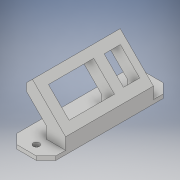
# Autodesk Inventor part: Indicator
Saved by Autodesk Inventor 2019.4 (Build 234330000, 330)
## iProperties
Created: 2020-04-10
Part Number: Indicator
Material: Типовые
Document SubType Name: Modeling
Designer: NoName
Density: 1 g/cm^3
Appearance: По умолчанию
Author: NoName
Autodesk Inventor part; units mm, degrees
ref_plane "YZ Plane" through (0, 0, 0) normal (1, 0, 0) x (0, 1, 0)
ref_plane "XZ Plane" through (0, 0, 0) normal (0, 1, 0) x (-1, 0, 0)
ref_plane "XY Plane" through (0, 0, 0) normal (0, 0, 1) x (1, 0, 0)
sketch "Эскиз1" plane through (0, 0, 0) normal (0, 0, 1) x (1, 0, 0)
  line L0 (-10, 0) -> (10, 0)
  line L1 (-10, 25) -> (-10, 0)
  line L2 (-10, 25) -> (-7, 25)
  line L3 (-7, 25) -> (10, 8)
  line L4 (10, 8) -> (10, 0)
  point P0 (0, 0)
  point P1 (0, 0)
  dimension "d4" = 20
  dimension "d5" = 25
  dimension "d6" = 3
  dimension "d7" = 135
  constraints: 10 end point, 2 horizontal, 1 coincident, 1 midpoint, 1 perpendicular
  measures "d4" distance of L0.start L0.end
  measures "d5" distance of L1.start L0.start
  measures "d6" distance of L1.start L2.end
  measures "d7" angle of L4 L3
extrude "Выдавливание1" add sketch "Эскиз1" along normal mid plane 45
sketch "Эскиз3" plane through (-7, 25, -22.5) normal (0.7071, 0.7071, 0) x (-0.7071, 0.7071, 0)
  line L0 (-4.5208, 40) -> (-19.5208, 40)
  line L1 (-19.5208, 40) -> (-19.5208, 16.8)
  line L2 (-19.5208, 16.8) -> (-4.5208, 16.8)
  line L3 (-4.5208, 16.8) -> (-4.5208, 40)
  line L4 (-24.0416, 45) -> (0, 45) projected
  line L5 (-5.0208, 11.8) -> (-19.0208, 11.8)
  line L6 (-19.0208, 11.8) -> (-19.0208, 3.5)
  line L7 (-19.0208, 3.5) -> (-5.0208, 3.5)
  line L8 (-5.0208, 3.5) -> (-5.0208, 11.8)
  line L9 (0, 0) -> (-24.0416, 0) projected
  point P0 (-22.6274, 22.5)
  point P1 (-12.0208, 11.8)
  point P2 (-12.0208, 16.8)
  point P3 (-12.0208, 3.5)
  point P4 (-12.0208, 0)
  dimension "d8" = 23.2
  dimension "d9" = 15
  dimension "d10" = 5
  dimension "d11" = 14
  dimension "d12" = 8.3
  dimension "d13" = 5
  constraints: 16 end point, 4 midpoint, 4 parallel, 2 horizontal, 2 perpendicular, 2 vertical alignment
  measures "d8" distance between parallel lines of L2 L0
  measures "d9" distance between parallel lines of L1 L3
  measures "d10" distance between parallel lines of L4 L0
  measures "d11" distance of L6.end L7.end
  measures "d12" distance of L7.end L5.start
  measures "d13" distance between parallel lines of L2 L5
extrude "Выдавливание2" cut sketch "Эскиз3" against normal blind 10
sketch "Эскиз7" plane through (0, 0, 22.5) normal (0, 0, 1) x (1, 0, 0)
  line L0 (10, 0) -> (-10, 0) projected
  line L1 (0, 8.1005) -> (-10, 18.1005)
  line L2 (10, 8) -> (-7, 25) projected
  line L3 (6.8033, 11.1967) -> (-3.8033, 21.8033) projected
  line L4 (10, 8) -> (10, 0) projected
  line L5 (-7, 25) -> (10, 8)
  line L6 (-7, 25) -> (10, 8) projected
  line L7 (0, 8.1005) -> (0, 2)
  line L8 (0, 2) -> (-10, 2)
  line L9 (-10, 2) -> (-10, 0)
  line L10 (-10, 0) -> (10, 0)
  line L11 (10, 8) -> (10, 0)
  line L12 (-10, 18.1005) -> (-10, 22)
  line L13 (-10, 22) -> (-7, 25)
  line L14 (-10, 25) -> (-10, 0) projected
  point P0 (0, 0)
  point P1 (1.5, 16.5)
  dimension "d22" = 7
  dimension "d24" = 2
  dimension "d25" = 10
  dimension "d26" = 135
  constraints: 18 end point, 3 vertical, 2 collinear, 1 midpoint, 1 parallel, 1 point on line
  measures "d22" distance between parallel lines of L2 L1
  measures "d24" distance between parallel lines of L0 L8
  measures "d25" distance between parallel lines of L4 L7
  measures "d26" angle of L12 L13
extrude "Выдавливание4" cut sketch "Эскиз7" against normal through all contours L0 L9 L8 L7 L1 L12 L13 L2 L4 keep common part
sketch "Эскиз8" plane through (0, 0, -22.5) normal (0, 0, -1) x (-1, 0, 0)
  line L0 (10, 2) -> (0, 2) projected
  line L1 (-10, 0) -> (10, 0) projected
  line L2 (10, 2) -> (-10, 2)
  line L3 (-10, 2) -> (-10, 0)
  line L4 (-10, 0) -> (10, 0)
  line L5 (10, 0) -> (10, 2)
  point P0 (0, 0)
  constraints: 8 end point, 2 parallel, 1 horizontal, 1 perpendicular
extrude "Выдавливание5" add sketch "Эскиз8" along normal blind 10
chamfer "Фаска1" distance 5 angle 45 2 edges at (10, 1, -32.5) (-10, 1, -32.5)
mirror "Зеркальное отражение1" about plane through (0, 0, 0) normal (0, 0, 1) of "Выдавливание5", "Фаска1"
sketch "Эскиз9" plane through (0, 2, 22.5) normal (0, 1, 0) x (1, 0, 0)
  line L0 (10, 0) -> (-7, 0) projected
  line L1 (0, 0) -> (0, 45) projected
  point P0 (0, 22.5)
  point P1 (0, 50)
  point P2 (0, -5)
  point P3 (0, 22.5)
  dimension "d41" = 55
  dimension "d42" = 5
  constraints: 2 vertical alignment, 1 midpoint
  measures "d41" distance of point (0, -5) point (0, 50)
  measures "d42" distance from line of L0 point (0, -5)
hole "Отверстие1" at (0, 2, -27.5) at (0, 2, 27.5) direction (0, -1, 0) diameter 3.2 end through all
